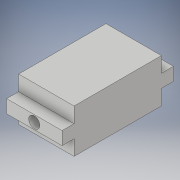
# Autodesk Inventor part: FrameSpacer
Saved by Autodesk Inventor 2017 (Build 210142000, 142)
## iProperties
Created: 2017-09-23
Part Number: FrameSpacer
Material: Generic
Document SubType Name: Modeling
Designer: User
Density: 1 g/cm^3
Appearance: Default
Author: User
Autodesk Inventor part; units mm, degrees
ref_plane "YZ Plane" through (0, 0, 0) normal (1, 0, 0) x (0, 1, 0)
ref_plane "XZ Plane" through (0, 0, 0) normal (0, 1, 0) x (-1, 0, 0)
ref_plane "XY Plane" through (0, 0, 0) normal (0, 0, 1) x (1, 0, 0)
sketch "Sketch1" plane through (0, 0, 0) normal (1, 0, 0) x (0, 1, 0)
  line L0 (20, 0) -> (20, -40.0304)
  line L1 (20, -40.0304) -> (0, -40.0304)
  line L2 (0, -40.0304) -> (0, 0)
  line L3 (12.9972, 0) -> (7.0028, 0)
  line L4 (7.0028, 0) -> (7.0028, 5.5118)
  line L5 (7.0028, 5.5118) -> (12.9972, 5.5118)
  line L6 (12.9972, 5.5118) -> (12.9972, 0)
  line L7 (12.9972, -40.0304) -> (7.0028, -40.0304)
  line L8 (7.0028, -40.0304) -> (7.0028, -45.5422)
  line L9 (7.0028, -45.5422) -> (12.9972, -45.5422)
  line L10 (12.9972, -45.5422) -> (12.9972, -40.0304)
  line L11 (0, 0) -> (7.0028, 0)
  line L12 (12.9972, 0) -> (20, 0)
  dimension "d0" = 20
  dimension "d1" = 40.0304
  dimension "d2" = 5.5118
  dimension "d3" = 5.9944
  dimension "d4" = 5.5118
  dimension "d5" = 7.0028
  dimension "d6" = 7.0028
  dimension "d7" = 5.9944
  constraints: 26 end point, 7 parallel, 4 horizontal, 4 perpendicular, 1 point on line
  measures "d0" distance of L0.end L1.end
  measures "d1" distance of L0.start L0.end
  measures "d2" distance of L3.end L4.end
  measures "d3" distance of L4.end L5.end
  measures "d4" distance of L7.end L8.end
  measures "d5" distance between parallel lines of L0 L6
  measures "d6" distance between parallel lines of L0 L10
  measures "d7" distance of L8.end L9.end
extrude "Extrusion1" add sketch "Sketch1" along normal blind 25.4
sketch "Sketch2" plane through (0, 7.0028, 5.5118) normal (0, 0, 1) x (1, 0, 0)
  line L0 (0, 5.9944) -> (25.4, 5.9944) projected
  line L1 (25.4, 12.9972) -> (25.4, 5.9944) projected
  line L2 (0, 12.9972) -> (25.4, 12.9972) projected
  line L3 (0, 12.9972) -> (0, 5.9944) projected
  line L4 (0, 5.9944) -> (0, 0) projected
  line L5 (0, 0) -> (25.4, 0) projected
  line L6 (25.4, 5.9944) -> (25.4, 0) projected
  line L7 (0, 5.9944) -> (25.4, 5.9944) projected
  line L8 (0, 0) -> (25.4, 0) projected
  line L9 (0, 0) -> (0, -7.0028) projected
  line L10 (0, -7.0028) -> (25.4, -7.0028) projected
  line L11 (25.4, 0) -> (25.4, -7.0028) projected
  circle A0 centre (12.7, 2.9972) radius 2.54
  dimension "d10" = 5.08
  constraints: 1 centre point
  measures "d10" diameter of A0
extrude "Extrusion2" cut sketch "Sketch2" against normal blind 127 contours A0
equation "\"d4\" = d2"
equation "\"d5\" = 0.5 * d0 - 0.5 * d3"
equation "\"d6\" = d5"
equation "\"d7\" = d3"
body "Solid1"
